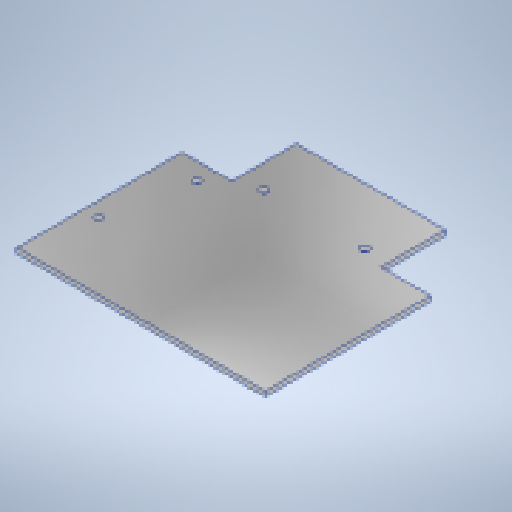
# Autodesk Inventor part: minisumopodsr
Saved by Autodesk Inventor 2023 (Build 270158000, 158)
## iProperties
Created: 2022-10-10
Part Number: minisumopodsr
Material: Aluminum 6061
Document SubType Name: Modeling
Designer: komputer
Density: 2.7 g/cm^3
Appearance: Aluminum - Flat
Author: komputer
Autodesk Inventor part; units mm, degrees
ref_plane "YZ Plane" through (0, 0, 0) normal (1, 0, 0) x (0, 1, 0)
ref_plane "XZ Plane" through (0, 0, 0) normal (0, 1, 0) x (-1, 0, 0)
ref_plane "XY Plane" through (0, 0, 0) normal (0, 0, 1) x (1, 0, 0)
sketch "Sketch1" plane through (0, 0, 0) normal (0, 1, 0) x (-1, 0, 0)
  line L0 (-95.7688, 101.9192) -> (4.2312, 101.9192)
  line L1 (4.2312, 101.9192) -> (4.2312, 1.9192)
  line L2 (4.2312, 1.9192) -> (-95.7688, 1.9192)
  line L3 (-95.7688, 1.9192) -> (-95.7688, 101.9192)
  line L4 (-95.7688, 1.9192) -> (4.2312, 1.9192)
  line L5 (4.2312, 1.9192) -> (4.2312, 6.9192)
  line L6 (4.2312, 6.9192) -> (-95.7688, 6.9192)
  line L7 (-95.7688, 6.9192) -> (-95.7688, 1.9192)
  line L8 (4.2312, 1.9192) -> (-15.7688, 1.9192)
  line L9 (-15.7688, 1.9192) -> (-15.7688, 32.9192)
  line L10 (-15.7688, 32.9192) -> (4.2312, 32.9192)
  line L11 (4.2312, 32.9192) -> (4.2312, 1.9192)
  line L12 (-95.7688, 1.9192) -> (-75.7688, 1.9192)
  line L13 (-75.7688, 1.9192) -> (-75.7688, 32.9192)
  line L14 (-75.7688, 32.9192) -> (-95.7688, 32.9192)
  line L15 (-95.7688, 32.9192) -> (-95.7688, 1.9192)
  point P0 (0, 0)
  dimension "d0" = 100
  dimension "d1" = 100
  dimension "d2" = 5
  dimension "d3" = 20
  dimension "d4" = 31
  dimension "d5" = 20
  constraints: 32 end point, 8 parallel, 4 horizontal, 4 perpendicular, 2 point on line
  measures "d0" distance of L1.end L2.end
  measures "d1" distance of L0.end L1.end
  measures "d2" distance of L5.end L4.end
  measures "d3" distance of L9.end L10.end
  measures "d4" distance of L8.end L9.end
  measures "d5" distance of L14.end L13.end
extrude "Extrusion1" add sketch "Sketch1" along normal blind 2 contours L0 L1 L10 L9 L6 L13 L14 L3 | L6 L9 L2 L13
sketch "Sketch2" plane through (0, 2, 0) normal (0, 1, 0) x (1, 0, 0)
  line L0 (-4.2312, -82.6348) -> (-4.2312, -11.6268) projected
  line L1 (95.7688, -11.6268) -> (95.7688, -82.6348) projected
  line L2 (75.7688, -32.9192) -> (75.7688, -1.9192) projected
  line L3 (15.7688, -1.9192) -> (15.7688, -32.9192) projected
  line L4 (75.7688, -1.9192) -> (15.7688, -1.9192)
  line L5 (15.7688, -1.9192) -> (15.7688, -6.9192)
  line L6 (15.7688, -6.9192) -> (75.7688, -6.9192)
  line L7 (75.7688, -6.9192) -> (75.7688, -1.9192)
  line L8 (95.7688, -82.6348) -> (-4.2312, -82.6348) projected
  line L9 (95.7688, -11.6268) -> (-4.2312, -11.6268) projected
  point P0 (0, 0)
  dimension "d8" = 5
  constraints: 8 end point, 2 parallel, 1 horizontal, 1 perpendicular, 1 point on line
  measures "d8" distance of L5.end L4.end
extrude "Extrusion2" cut sketch "Sketch2" against normal blind 2 contours L3 L4 L2 L6
sketch "Szkic3" plane through (0, 2, 0) normal (0, 1, 0) x (1, 0, 0)
  circle A0 centre (66.0188, -29.6192) radius 1.75
  circle A1 centre (25.5188, -29.6192) radius 1.75
  point P0 (0, 0)
  constraints: 2 centre point, 4 other
extrude "Wyciągnięcie proste3" cut sketch "Szkic3" against normal through all
sketch "Szkic4" plane through (0, 0, 0) normal (0, -1, 0) x (1, 0, 0)
  circle A0 centre (25.5188, 29.6192) radius 1.75 projected
  circle A1 centre (66.0188, 29.6192) radius 1.75 projected
  line L0 (15.7688, 6.9192) -> (75.7688, 6.9192) projected
  line L1 (75.7688, 32.9192) -> (75.7688, 6.9192) projected
  line L2 (95.7688, 32.9192) -> (75.7688, 32.9192) projected
  line L3 (95.7688, 101.9192) -> (95.7688, 32.9192) projected
  line L4 (-4.2312, 101.9192) -> (95.7688, 101.9192) projected
  line L5 (-4.2312, 32.9192) -> (-4.2312, 101.9192) projected
  line L6 (15.7688, 32.9192) -> (-4.2312, 32.9192) projected
  line L7 (15.7688, 6.9192) -> (15.7688, 32.9192) projected
  point P0 (0, 0)
extrude "Wyciągnięcie proste4" add sketch "Szkic4" against normal up to surface (2 mm away) contours A0 | A1
sketch "Szkic5" plane through (0, 2, 0) normal (0, 1, 0) x (1, 0, 0)
  circle A0 centre (22.8938, -32.6829) radius 1.5
  circle A1 centre (68.6438, -32.6829) radius 1.5
  point P0 (0, 0)
  constraints: 2 centre point, 4 other
extrude "Wyciągnięcie proste5" cut sketch "Szkic5" against normal through all
sketch "Szkic6" plane through (-4.2312, 0, 101.9192) normal (0, 0, 1) x (1, 0, 0)
  line L0 (0, 0) -> (100, 0) projected
  line L1 (100, 0) -> (100, 2) projected
  line L2 (0, 2) -> (100, 2) projected
  line L3 (0, 0) -> (0, 2) projected
  point P0 (4.2312, 0)
extrude "Wyciągnięcie proste6" cut sketch "Szkic6" against normal blind 2.5
sketch "Szkic7" plane through (0, 0, 0) normal (0, -1, 0) x (1, 0, 0)
  circle A0 centre (1.7688, 72.4703) radius 1.5
  circle A1 centre (8.7688, 39.9192) radius 1.5
  point P0 (0, 0)
  constraints: 2 centre point, 4 other
extrude "Wyciągnięcie proste7" cut sketch "Szkic7" against normal through all
sketch "Szkic8" plane through (0, 0, 0) normal (0, -1, 0) x (1, 0, 0)
  circle A0 centre (8.7688, 39.9192) radius 1.5 projected
  circle A1 centre (1.7688, 72.4703) radius 1.5 projected
  line L0 (95.7688, 99.4192) -> (-4.2312, 99.4192) projected
  line L1 (-4.2312, 32.9192) -> (-4.2312, 99.4192) projected
  line L2 (15.7688, 32.9192) -> (-4.2312, 32.9192) projected
  line L3 (15.7688, 6.9192) -> (15.7688, 32.9192) projected
  line L4 (15.7688, 6.9192) -> (75.7688, 6.9192) projected
  line L5 (75.7688, 32.9192) -> (75.7688, 6.9192) projected
  line L6 (95.7688, 32.9192) -> (75.7688, 32.9192) projected
  line L7 (95.7688, 99.4192) -> (95.7688, 32.9192) projected
  circle A2 centre (22.8938, 32.6829) radius 1.5 projected
  circle A3 centre (68.6438, 32.6829) radius 1.5 projected
  line L8 (-4.2312, 39.9192) -> (21.3688, 39.9192)
  circle A4 centre (21.3688, 39.9192) radius 2.1391
  line L9 (-4.2312, 32.9192) -> (-4.2312, 60.9192)
  line L10 (-4.2312, 32.9192) -> (-4.2312, 99.4192) projected
  point P0 (0, 0)
  dimension "d21" = 25.6
  dimension "d22" = 28
  constraints: 4 end point, 2 point on line, 1 centre point, 1 coincident, 1 horizontal
  measures "d21" distance of L8.start L8.end
  measures "d22" distance of L1.start L9.end
sketch "Szkic9" plane through (0, 0, 0) normal (0, -1, 0) x (1, 0, 0)
  circle A0 centre (25.5188, 29.6192) radius 1.75
  circle A1 centre (66.0188, 29.6192) radius 1.75
  point P0 (0, 0)
  constraints: 2 centre point, 4 other
extrude "Wyciągnięcie proste8" cut sketch "Szkic9" against normal through all
extrude "Wyciągnięcie proste9" add sketch "Szkic8" against normal up to surface (2 mm away) contours A2 | A3
sketch "Szkic10" plane through (0, 0, 0) normal (0, -1, 0) x (1, 0, 0)
  circle A0 centre (45.7688, 11.3479) radius 1.5
  point P0 (0, 0)
  constraints: 1 centre point, 2 other
extrude "Wyciągnięcie proste10" cut sketch "Szkic10" against normal through all
body "Solid1"
